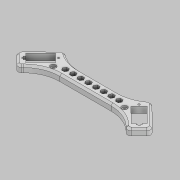
# Autodesk Inventor part: Chassis_V2
Saved by Autodesk Inventor 2022.2 (Build 262287010, 287A)
## iProperties
Created: 2022-06-14
Part Number: Chassis_V2
Material: Genérico
Document SubType Name: Modeling
Designer: Usuario
Density: 1 g/cm^3
Appearance: Valor por defecto
Author: Usuario
Autodesk Inventor part; units mm, degrees
ref_plane "YZ Plane" through (0, 0, 0) normal (1, 0, 0) x (0, 1, 0)
ref_plane "XZ Plane" through (0, 0, 0) normal (0, 1, 0) x (-1, 0, 0)
ref_plane "XY Plane" through (0, 0, 0) normal (0, 0, 1) x (1, 0, 0)
sketch "Boceto1" plane through (0, 0, 0) normal (0, 1, 0) x (-1, 0, 0)
  line L0 (0, -15) -> (37.8285, -15)
  line L1 (0, 0) -> (44.5466, 0)
  line L2 (59.8775, 15.2884) -> (74, 1.1266)
  line L3 (74, 1.1266) -> (47.8008, -25)
  line L4 (47.8008, -25) -> (37.8285, -15)
  line L5 (33.6783, -10.8383) -> (44.5466, 0) construction
  line L6 (59.8775, 15.2884) -> (39.8775, 15.2884) construction
  circle A0 centre (39, -3.8) radius 1.5
  line L7 (37.8285, -15) -> (33.6783, -10.8383) construction
  line L8 (44.5466, 0) -> (59.8775, 15.2884)
  line L9 (0, 0) -> (0, 6.3504) construction
  line L10 (0, 0) -> (0, -23.2363) construction
  line L11 (0, -15) -> (-37.8285, -15)
  line L12 (0, 0) -> (-44.5466, 0)
  line L13 (-59.8775, 15.2884) -> (-74, 1.1266)
  line L14 (-74, 1.1266) -> (-47.8008, -25)
  line L15 (-47.8008, -25) -> (-37.8285, -15)
  line L16 (-33.6783, -10.8383) -> (-44.5466, 0) construction
  circle A1 centre (-39, -3.8) radius 1.5
  line L17 (-37.8285, -15) -> (-33.6783, -10.8383) construction
  line L18 (-44.5466, 0) -> (-59.8775, 15.2884)
  dimension "d1" = 10
  dimension "d2" = 15
  dimension "d4" = 20
  dimension "d5" = 37
  dimension "d6" = 0
  dimension "d7" = 3
  dimension "d10" = 3.8
  dimension "d11" = 39
  constraints: 38 end point, 7 symmetric about line, 4 parallel, 3 horizontal, 2 centre point, 2 vertical, 1 equal length, 1 perpendicular, 1 other
  measures "d1" distance from line of L0 L3.end
  measures "d2" distance between parallel lines of L1 L0
  measures "d4" distance between parallel lines of L3 L5
  measures "d5" distance of L2.end L3.end
  measures "d6" horizontal distance of L0.start L1.start
  measures "d7" diameter of A0
  measures "d10" distance from line of L1 A0.centre
  measures "d11" horizontal distance of L1.start A0.centre
extrude "Extrusión1" add sketch "Boceto1" along normal blind 7
fillet "Empalme1" radius 40 4 edges at (-37.8285, 3.5, -15) (37.8285, 3.5, -15) (-44.5466, 3.5, 0) (44.5466, 3.5, 0)
sketch "Boceto2" plane through (0, 7, 0) normal (0, 1, 0) x (1, 0, 0)
  line L0 (0, 0) -> (0, -9.3578) construction
  line L1 (-2.6123, 4.75) -> (-5.7877, 4.75)
  line L2 (-5.7877, 4.75) -> (-7.3754, 7.5)
  line L3 (-7.3754, 7.5) -> (-5.7877, 10.25)
  line L4 (-5.7877, 10.25) -> (-2.6123, 10.25)
  line L5 (-2.6123, 10.25) -> (-1.0246, 7.5)
  line L6 (-1.0246, 7.5) -> (-2.6123, 4.75)
  line L7 (21.3433, 15) -> (-21.3433, 15) projected
  line L8 (-28.0106, 0) -> (28.0106, 0) projected
  line L9 (-14.1877, 10.25) -> (-11.0123, 10.25)
  line L10 (-15.7754, 7.5) -> (-14.1877, 10.25)
  line L11 (-14.1877, 4.75) -> (-15.7754, 7.5)
  line L12 (-11.0123, 4.75) -> (-14.1877, 4.75)
  line L13 (-9.4246, 7.5) -> (-11.0123, 4.75)
  line L14 (-11.0123, 10.25) -> (-9.4246, 7.5)
  line L15 (-22.5877, 10.25) -> (-19.4123, 10.25)
  line L16 (-24.1754, 7.5) -> (-22.5877, 10.25)
  line L17 (-22.5877, 4.75) -> (-24.1754, 7.5)
  line L18 (-19.4123, 4.75) -> (-22.5877, 4.75)
  line L19 (-17.8246, 7.5) -> (-19.4123, 4.75)
  line L20 (-19.4123, 10.25) -> (-17.8246, 7.5)
  line L21 (-30.9877, 10.25) -> (-27.8123, 10.25)
  line L22 (-32.5754, 7.5) -> (-30.9877, 10.25)
  line L23 (-30.9877, 4.75) -> (-32.5754, 7.5)
  line L24 (-27.8123, 4.75) -> (-30.9877, 4.75)
  line L25 (-26.2246, 7.5) -> (-27.8123, 4.75)
  line L26 (-27.8123, 10.25) -> (-26.2246, 7.5)
  line L27 (2.6123, 4.75) -> (5.7877, 4.75)
  line L28 (5.7877, 4.75) -> (7.3754, 7.5)
  line L29 (7.3754, 7.5) -> (5.7877, 10.25)
  line L30 (5.7877, 10.25) -> (2.6123, 10.25)
  line L31 (2.6123, 10.25) -> (1.0246, 7.5)
  line L32 (1.0246, 7.5) -> (2.6123, 4.75)
  line L33 (14.1877, 10.25) -> (11.0123, 10.25)
  line L34 (15.7754, 7.5) -> (14.1877, 10.25)
  line L35 (14.1877, 4.75) -> (15.7754, 7.5)
  line L36 (11.0123, 4.75) -> (14.1877, 4.75)
  line L37 (9.4246, 7.5) -> (11.0123, 4.75)
  line L38 (11.0123, 10.25) -> (9.4246, 7.5)
  line L39 (22.5877, 10.25) -> (19.4123, 10.25)
  line L40 (24.1754, 7.5) -> (22.5877, 10.25)
  line L41 (22.5877, 4.75) -> (24.1754, 7.5)
  line L42 (19.4123, 4.75) -> (22.5877, 4.75)
  line L43 (17.8246, 7.5) -> (19.4123, 4.75)
  line L44 (19.4123, 10.25) -> (17.8246, 7.5)
  line L45 (30.9877, 10.25) -> (27.8123, 10.25)
  line L46 (32.5754, 7.5) -> (30.9877, 10.25)
  line L47 (30.9877, 4.75) -> (32.5754, 7.5)
  line L48 (27.8123, 4.75) -> (30.9877, 4.75)
  line L49 (26.2246, 7.5) -> (27.8123, 4.75)
  line L50 (27.8123, 10.25) -> (26.2246, 7.5)
  point P0 (-4.2, 7.5)
  point P1 (0, 0)
  point P2 (4.2, 7.5)
  dimension "d17" = 5.5
  dimension "d18" = 7.5
  dimension "d19" = 4.2
  dimension "d22" = 8.4
  constraints: 98 end point, 25 symmetric about line, 2 horizontal, 1 midpoint, 1 vertical, 49 other
  measures "d17" distance between parallel lines of L1 L4
  measures "d18" distance from line of point (-4.2, 7.5) L7
  measures "d19" horizontal distance of point (0, 0) point (-4.2, 7.5)
  measures "d22" distance of L3.end L9.start
extrude "Extrusión2" cut sketch "Boceto2" against normal up to surface (7 mm away)
sketch "Boceto4" plane through (0, 7, 0) normal (0, 1, 0) x (1, 0, 0)
  line L0 (-50.1094, 17.4018) -> (-41.2829, 8.5507)
  line L1 (-41.2829, 8.5507) -> (-57.5689, -7.6902)
  line L2 (-57.5689, -7.6902) -> (-66.3954, 1.1609)
  line L3 (-66.3954, 1.1609) -> (-50.1094, 17.4018)
  line L4 (-47.8008, 25) -> (-74, -1.1266) projected
  line L5 (-60.9004, 11.9367) -> (-64.3486, 15.3945) construction
  line L6 (-74, -1.1266) -> (-59.8775, -15.2884) projected
  line L7 (-66.9387, -8.2075) -> (-71.8609, -13.116) construction
  line L8 (0, 0) -> (0, -9.0958) construction
  line L9 (50.1094, 17.4018) -> (41.2829, 8.5507)
  line L10 (41.2829, 8.5507) -> (57.5689, -7.6902)
  line L11 (57.5689, -7.6902) -> (66.3954, 1.1609)
  line L12 (66.3954, 1.1609) -> (50.1094, 17.4018)
  dimension "d32" = 12.5
  dimension "d33" = 23
  constraints: 22 end point, 6 symmetric about line, 3 perpendicular, 2 midpoint, 2 parallel, 1 vertical
  measures "d32" distance of L0.start L0.end
  measures "d33" distance of L0.end L1.end
extrude "Extrusión3" cut sketch "Boceto4" against normal up to surface (7 mm away)
sketch "Boceto5" plane through (0, 7, 0) normal (0, 1, 0) x (1, 0, 0)
  circle A0 centre (-39, 3.8) radius 1.5 projected
  circle A1 centre (39, 3.8) radius 1.5 projected
  circle A2 centre (-39, 3.8) radius 3
  circle A3 centre (39, 3.8) radius 3
  point P0 (0, 0)
  dimension "d36" = 6
  dimension "d37" = 6
  constraints: 2 centre point, 2 coincident
  measures "d36" diameter of A2
  measures "d37" diameter of A3
extrude "Extrusión4" cut sketch "Boceto5" against normal blind 2 contours A0 | A1 | A2 | A3
sketch "Boceto6" plane through (0, 7, 0) normal (0, 1, 0) x (1, 0, 0)
  line L0 (-66.9387, -8.2075) -> (-68.11, -9.3755) construction
  line L1 (-59.8163, 2.0728) -> (-56.6387, -1.1136)
  line L2 (-56.6387, -1.1136) -> (-61.8095, -6.2701)
  line L3 (-61.8095, -6.2701) -> (-64.9871, -3.0837)
  line L4 (-64.9871, -3.0837) -> (-59.8163, 2.0728)
  line L5 (-57.5689, -7.6902) -> (-66.3954, 1.1609) projected
  line L6 (0, 0) -> (0, -8.3332) construction
  line L7 (59.8163, 2.0728) -> (56.6387, -1.1136)
  line L8 (56.6387, -1.1136) -> (61.8095, -6.2701)
  line L9 (61.8095, -6.2701) -> (64.9871, -3.0837)
  line L10 (64.9871, -3.0837) -> (59.8163, 2.0728)
  dimension "d44" = 4.5
  dimension "d45" = 2
  constraints: 20 end point, 5 symmetric about line, 2 parallel, 1 perpendicular, 1 vertical
  measures "d44" distance of L1.start L1.end
  measures "d45" distance between parallel lines of L3 L5
extrude "Extrusión5" cut sketch "Boceto6" against normal up to surface (7 mm away)
sketch "Boceto7" plane through (0, 7, 0) normal (0, 1, 0) x (1, 0, 0)
  circle A0 centre (-44.0321, 14.6356) radius 1
  circle A1 centre (-63.6461, -4.924) radius 1
  line L0 (-47.8008, 25) -> (-74, -1.1266) projected
  line L1 (-60.9004, 11.9367) -> (-64.4807, 15.5269) construction
  line L2 (-41.2829, 8.5507) -> (-57.5689, -7.6902) projected
  line L3 (0, 0) -> (0, -6.643) construction
  circle A2 centre (44.0321, 14.6356) radius 1
  circle A3 centre (63.6461, -4.924) radius 1
  dimension "d48" = 2
  dimension "d49" = 2
  dimension "d50" = 27.7
  dimension "d51" = 6.25
  constraints: 4 centre point, 4 end point, 3 symmetric about line, 1 midpoint, 1 perpendicular, 1 vertical, 2 other
  measures "d48" diameter of A0
  measures "d49" diameter of A1
  measures "d50" distance of A1.centre A0.centre
  measures "d51" distance from line of L2 A0.centre
extrude "Extrusión6" cut sketch "Boceto7" against normal up to surface (7 mm away)
fillet "Empalme3" radius 4 6 edges at (-59.8775, 3.5, 15.2884) (-74, 3.5, 1.1266) (59.8775, 3.5, 15.2884) (74, 3.5, 1.1266) (-47.8008, 3.5, -25) (47.8008, 3.5, -25)
chamfer "Chaflán2" distance 2 angle 45 18 edges at (-33.8714, 7, -17.0126) (0, 7, -15) (33.8714, 7, -17.0126) (47.812, 7, -23.6217) (60.7553, 7, -12.0814) (72.3431, 7, 1.1289) (66.9387, 7, 8.2075) (59.8752, 7, 13.6315) (56.6504, 7, 12.0702) (43.2923, 7, 3.0342) (0, 7, 0) (-43.2923, 7, 3.0342) (-56.6504, 7, 12.0702) (-59.8752, 7, 13.6315) (-66.9387, 7, 8.2075) (-72.3431, 7, 1.1289) (-60.7553, 7, -12.0814) (-47.812, 7, -23.6217)
